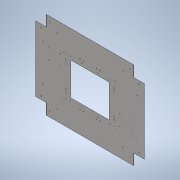
# Autodesk Inventor part: Chapa-0001-002
Saved by Autodesk Inventor 2020.1 (Build 241239000, 239)
## iProperties
Created: 2024-04-13
Part Number: Chapa-0001-002
Material: Steel, Galvanized
Document SubType Name: Sheet Metal
Designer: MiguelBarbosa
Density: 7.85 g/cm^3
Sheet Metal Rule: Default_mm
Appearance: Galvanized
Author: MiguelBarbosa
Autodesk Inventor part; units mm, degrees
ref_plane "YZ Plane" through (0, 0, 0) normal (1, 0, 0) x (0, 1, 0)
ref_plane "XZ Plane" through (0, 0, 0) normal (0, 1, 0) x (-1, 0, 0)
ref_plane "XY Plane" through (0, 0, 0) normal (0, 0, 1) x (1, 0, 0)
sketch "Sketch1" plane through (0, 0, 0) normal (0, 0, 1) x (1, 0, 0)
  line L0 (-500, -400) -> (500, -400)
  line L1 (500, -400) -> (500, 400)
  line L2 (500, 400) -> (-500, 400)
  line L3 (-500, 400) -> (-500, -400)
  line L4 (-500, -400) -> (500, 400) construction
  line L5 (500, -400) -> (-500, 400) construction
  point P0 (0, 0)
  dimension "d0" = 1000
  dimension "d1" = 800
  measures "d0" distance of L1.end L2.end
  measures "d1" distance of L2.end L0.start
extrude "Plate1" add sketch "Sketch1" along normal mid plane 0.5
sketch "Sketch2" plane through (0, 0, 0.25) normal (0, 0, 1) x (1, 0, 0)
  line L0 (-175, -150) -> (175, -150)
  line L1 (175, -150) -> (175, 150)
  line L2 (175, 150) -> (-175, 150)
  line L3 (-175, 150) -> (-175, -150)
  line L4 (-175, -150) -> (175, 150) construction
  line L5 (175, -150) -> (-175, 150) construction
  point P0 (0, 0)
  dimension "d3" = 350
  dimension "d4" = 300
  constraints: 12 end point, 2 midpoint, 2 parallel, 1 horizontal, 1 perpendicular
  measures "d3" distance of L1.end L2.end
  measures "d4" distance of L2.end L0.start
extrude "Cut1" cut sketch "Sketch2" against normal blind 0.5
sketch "Sketch3" plane through (0, 0, 0.25) normal (0, 0, 1) x (1, 0, 0)
  line L0 (-500, 300) -> (-400, 300)
  line L1 (-400, 300) -> (-400, 400)
  line L2 (-400, 400) -> (-500, 400)
  line L3 (-500, 400) -> (-500, 300)
  line L4 (-500, 300) -> (-400, 400) construction
  line L5 (-400, 300) -> (-500, 400) construction
  circle A0 centre (-450, 270) radius 5.1
  circle A1 centre (-370, 350) radius 5.1
  line L6 (-78.1, 171.9) -> (-71.9, 171.9)
  line L7 (-71.9, 171.9) -> (-71.9, 178.1)
  line L8 (-71.9, 178.1) -> (-78.1, 178.1)
  line L9 (-78.1, 178.1) -> (-78.1, 171.9)
  line L10 (-78.1, 171.9) -> (-71.9, 178.1) construction
  line L11 (-71.9, 171.9) -> (-78.1, 178.1) construction
  line L12 (-75, 175) -> (-75, 200) construction
  line L13 (-90, 200) -> (-60, 200) construction
  line L14 (-93.1, 196.9) -> (-86.9, 196.9)
  line L15 (-86.9, 196.9) -> (-86.9, 203.1)
  line L16 (-86.9, 203.1) -> (-93.1, 203.1)
  line L17 (-93.1, 203.1) -> (-93.1, 196.9)
  line L18 (-93.1, 196.9) -> (-86.9, 203.1) construction
  line L19 (-86.9, 196.9) -> (-93.1, 203.1) construction
  line L20 (-63.1, 196.9) -> (-56.9, 196.9)
  line L21 (-56.9, 196.9) -> (-56.9, 203.1)
  line L22 (-56.9, 203.1) -> (-63.1, 203.1)
  line L23 (-63.1, 203.1) -> (-63.1, 196.9)
  line L24 (-63.1, 196.9) -> (-56.9, 203.1) construction
  line L25 (-56.9, 196.9) -> (-63.1, 203.1) construction
  circle A2 centre (-430, 170) radius 5.1
  circle A3 centre (-300, 300) radius 5.1
  line L26 (-235, 180) -> (-225, 180) construction
  line L27 (-235, 174.9) -> (-225, 174.9)
  line L28 (-225, 185.1) -> (-235, 185.1)
  arc A4 (-235, 185.1) -> (-235, 174.9) centre (-235, 180) ccw
  arc A5 (-225, 174.9) -> (-225, 185.1) centre (-225, 180) ccw
  circle A6 centre (-180, 180) radius 5.1
  circle A7 centre (-220, 130) radius 5.1 construction
  circle A8 centre (-220, 100) radius 5.1 construction
  line L29 (-225.1, 124.9) -> (-214.9, 124.9)
  line L30 (-214.9, 124.9) -> (-214.9, 135.1)
  line L31 (-214.9, 135.1) -> (-225.1, 135.1)
  line L32 (-225.1, 135.1) -> (-225.1, 124.9)
  line L33 (-225.1, 124.9) -> (-214.9, 135.1) construction
  line L34 (-214.9, 124.9) -> (-225.1, 135.1) construction
  line L35 (-225.1, 94.9) -> (-214.9, 94.9)
  line L36 (-214.9, 94.9) -> (-214.9, 105.1)
  line L37 (-214.9, 105.1) -> (-225.1, 105.1)
  line L38 (-225.1, 105.1) -> (-225.1, 94.9)
  line L39 (-225.1, 94.9) -> (-214.9, 105.1) construction
  line L40 (-214.9, 94.9) -> (-225.1, 105.1) construction
  point P0 (0, 0)
  point P1 (-450, 350)
  point P2 (-450, 350)
  point P3 (-450, 350)
  point P4 (-230, 180)
  dimension "d7" = 100
  dimension "d10" = 10.2
  dimension "d11" = 30
  dimension "d12" = 30
  dimension "d30" = 175
  dimension "d31" = 75
  dimension "d32" = 6.2
  dimension "d33" = 25
  dimension "d34" = 30
  dimension "d38" = 430
  dimension "d39" = 170
  dimension "d40" = 10.2
  dimension "d44" = 300
  dimension "d45" = 300
  dimension "d46" = 10.2
  dimension "d47" = 230
  dimension "d48" = 180
  dimension "d49" = 10
  dimension "d50" = 10.2
  dimension "d52" = 180
  dimension "d53" = 180
  dimension "d54" = 10.2
  dimension "d59" = 220
  dimension "d60" = 30
  dimension "d61" = 10.2
  dimension "d62" = 100
  constraints: 84 end point, 16 midpoint, 13 parallel, 9 centre point, 8 horizontal, 8 tangent, 6 equal length, 6 perpendicular, 4 point on circle, 2 equal radius, 2 vertical alignment, 1 coincident, 1 horizontal alignment, 1 vertical
  measures "d7" distance of L0.start L0.end
  measures "d10" diameter of A0
  measures "d11" distance from line of A0.centre L0
  measures "d12" distance from line of A1.centre L1
  measures "d30" vertical distance of point (0, 0) L12.start
  measures "d31" horizontal distance of point (0, 0) L12.start
  measures "d32" distance of L7.end L8.end
  measures "d33" distance of L12.end L12.start
  measures "d34" distance of L13.start L13.end
  measures "d38" horizontal distance of point (0, 0) A2.centre
  measures "d39" vertical distance of point (0, 0) A2.centre
  measures "d40" diameter of A2
  measures "d44" horizontal distance of point (0, 0) A3.centre
  measures "d45" horizontal distance of point (0, 0) A3.centre
  measures "d46" diameter of A3
  measures "d47" horizontal distance of point (0, 0) point (-230, 180)
  measures "d48" vertical distance of point (0, 0) point (-230, 180)
  measures "d49" distance of L26.start L26.end
  measures "d50" distance between parallel lines of L27 L28
  measures "d52" horizontal distance of point (0, 0) A6.centre
  measures "d53" horizontal distance of point (0, 0) A6.centre
  measures "d54" diameter of A6
  measures "d59" horizontal distance of point (0, 0) A8.centre
  measures "d60" distance of A7.centre A8.centre
  measures "d61" diameter of A8
  measures "d62" vertical distance of point (0, 0) A8.centre
extrude "Cut2" cut sketch "Sketch3" against normal blind 0.5
mirror "Mirror1" about plane through (0, 0, 0) normal (1, 0, 0) of "Cut2"
mirror "Mirror2" about plane through (0, 0, 0) normal (0, 1, 0) of "Cut2", "Mirror1"
sketch "Sketch5" plane through (0, 0, 0.25) normal (0, 0, 1) x (1, 0, 0)
  circle A0 centre (-275, 150) radius 5.1
  circle A1 centre (-375, 150) radius 5.1
  circle A2 centre (-375, 50) radius 5.1
  circle A3 centre (-275, 50) radius 5.1
  line L0 (-375, 150) -> (-275, 150) construction
  line L1 (-275, 150) -> (-275, 50) construction
  line L2 (-275, 50) -> (-375, 50) construction
  line L3 (-375, 50) -> (-375, 150) construction
  line L4 (-375, 150) -> (-275, 50) construction
  line L5 (-275, 150) -> (-375, 50) construction
  line L6 (275, -50) -> (375, -50) construction
  line L7 (375, -50) -> (375, -150) construction
  line L8 (375, -150) -> (275, -150) construction
  line L9 (275, -150) -> (275, -50) construction
  line L10 (275, -50) -> (375, -150) construction
  line L11 (375, -50) -> (275, -150) construction
  circle A4 centre (275, -50) radius 5.1
  circle A5 centre (375, -50) radius 5.1
  circle A6 centre (275, -150) radius 5.1
  circle A7 centre (375, -150) radius 5.1
  point P0 (0, 0)
  point P1 (-325, 100)
  point P2 (325, -100)
  dimension "d18" = 10.2
  dimension "d19" = 325
  dimension "d20" = 100
  dimension "d21" = 100
  dimension "d22" = 100
  dimension "d23" = 100
  dimension "d24" = 325
  constraints: 24 end point, 8 centre point, 8 coincident, 7 equal radius, 6 parallel, 4 midpoint, 2 horizontal, 2 perpendicular
  measures "d18" diameter of A1
  measures "d19" horizontal distance of point (0, 0) point (-325, 100)
  measures "d20" vertical distance of point (0, 0) point (-325, 100)
  measures "d21" distance of L2.end L0.start
  measures "d22" distance of L0.start L0.end
  measures "d23" vertical distance of point (325, -100) point (0, 0)
  measures "d24" horizontal distance of point (0, 0) point (325, -100)
extrude "Cut4" cut sketch "Sketch5" against normal blind 0.5
equation "\"d5\" = Thickness"
equation "\"d12\" = d11"
equation "\"d8\" = Thickness"
equation "\"d22\" = d21"
equation "\"d23\" = d20"
equation "\"d24\" = d19"
equation "\"d25\" = Thickness"
equation "\"d2\" = Thickness"
equation "\"BendRadius\" = Thickness"
equation "\"BendReliefWidth\" = Thickness"
equation "\"BendReliefDepth\" = 0.5 * Thickness"
equation "\"CornerReliefSize\" = 4 * Thickness"
equation "\"MinimumRemnant\" = 2 * Thickness"
equation "\"TransitionRadius\" = BendRadius"
equation "\"JacobiRadiusSize\" = BendRadius"
equation "\"GapSize\" = Thickness"
equation "\"Thickness\" = 0.5"
body "Solid1"
